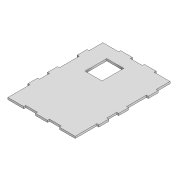
# Autodesk Inventor part: Sup´2
Saved by Autodesk Inventor 2022 (Build 260153000, 153)
## iProperties
Created: 2022-06-21
Part Number: Sup´2
Material: Generic
Document SubType Name: Modeling
Designer: ADMIN
Density: 1 g/cm^3
Appearance: Default
Author: ADMIN
Autodesk Inventor part; units mm, degrees
ref_plane "YZ Plane" through (0, 0, 0) normal (1, 0, 0) x (0, 1, 0)
ref_plane "XZ Plane" through (0, 0, 0) normal (0, 1, 0) x (-1, 0, 0)
ref_plane "XY Plane" through (0, 0, 0) normal (0, 0, 1) x (1, 0, 0)
sketch "Sketch1" plane through (0, 0, 0) normal (0, 1, 0) x (-1, 0, 0)
  line L0 (4.0305, 15.695) -> (174.0305, 15.695)
  line L1 (174.0305, 15.695) -> (174.0305, -224.305)
  line L2 (174.0305, -224.305) -> (4.0305, -224.305)
  line L3 (4.0305, -224.305) -> (4.0305, 15.695)
  line L4 (174.0305, -39.305) -> (169.0305, -39.305)
  line L5 (169.0305, -39.305) -> (169.0305, -64.305)
  line L6 (169.0305, -64.305) -> (174.0305, -64.305)
  line L7 (174.0305, -64.305) -> (174.0305, -39.305)
  line L8 (174.0305, -89.305) -> (169.0305, -89.305)
  line L9 (169.0305, -89.305) -> (169.0305, -114.305)
  line L10 (169.0305, -114.305) -> (174.0305, -114.305)
  line L11 (174.0305, -114.305) -> (174.0305, -89.305)
  line L12 (174.0305, -164.305) -> (169.0305, -164.305)
  line L13 (169.0305, -164.305) -> (169.0305, -189.305)
  line L14 (169.0305, -189.305) -> (174.0305, -189.305)
  line L15 (174.0305, -189.305) -> (174.0305, -164.305)
  line L16 (89.0305, 15.695) -> (89.0305, -224.305)
  line L17 (4.0305, -39.305) -> (9.0305, -39.305)
  line L18 (9.0305, -39.305) -> (9.0305, -64.305)
  line L19 (9.0305, -64.305) -> (4.0305, -64.305)
  line L20 (4.0305, -89.305) -> (9.0305, -89.305)
  line L21 (9.0305, -89.305) -> (9.0305, -114.305)
  line L22 (9.0305, -114.305) -> (4.0305, -114.305)
  line L23 (4.0305, -164.305) -> (9.0305, -164.305)
  line L24 (9.0305, -164.305) -> (9.0305, -189.305)
  line L25 (9.0305, -189.305) -> (4.0305, -189.305)
  line L26 (134.0305, 15.695) -> (104.0305, 15.695)
  line L27 (104.0305, 15.695) -> (104.0305, 10.695)
  line L28 (104.0305, 10.695) -> (134.0305, 10.695)
  line L29 (134.0305, 10.695) -> (134.0305, 15.695)
  line L30 (74.0305, 15.695) -> (44.0305, 15.695)
  line L31 (44.0305, 15.695) -> (44.0305, 10.695)
  line L32 (44.0305, 10.695) -> (74.0305, 10.695)
  line L33 (74.0305, 10.695) -> (74.0305, 15.695)
  line L34 (134.0305, -224.305) -> (104.0305, -224.305)
  line L35 (104.0305, -224.305) -> (104.0305, -219.305)
  line L36 (104.0305, -219.305) -> (134.0305, -219.305)
  line L37 (134.0305, -219.305) -> (134.0305, -224.305)
  line L38 (74.0305, -224.305) -> (44.0305, -224.305)
  line L39 (44.0305, -224.305) -> (44.0305, -219.305)
  line L40 (44.0305, -219.305) -> (74.0305, -219.305)
  line L41 (74.0305, -219.305) -> (74.0305, -224.305)
  line L42 (9.0305, -39.305) -> (-0.9695, -39.305)
  line L43 (-0.9695, -39.305) -> (-0.9695, -64.305)
  line L44 (-0.9695, -64.305) -> (9.0305, -64.305)
  line L45 (9.0305, -64.305) -> (9.0305, -39.305)
  line L46 (9.0305, -89.305) -> (-0.9695, -89.305)
  line L47 (-0.9695, -89.305) -> (-0.9695, -114.305)
  line L48 (-0.9695, -114.305) -> (9.0305, -114.305)
  line L49 (9.0305, -114.305) -> (9.0305, -89.305)
  line L50 (9.0305, -164.305) -> (-0.9695, -164.305)
  line L51 (-0.9695, -164.305) -> (-0.9695, -189.305)
  line L52 (-0.9695, -189.305) -> (9.0305, -189.305)
  line L53 (9.0305, -189.305) -> (9.0305, -164.305)
  line L54 (169.0305, -39.305) -> (179.0305, -39.305)
  line L55 (179.0305, -39.305) -> (179.0305, -64.305)
  line L56 (179.0305, -64.305) -> (169.0305, -64.305)
  line L57 (169.0305, -89.305) -> (179.0305, -89.305)
  line L58 (179.0305, -89.305) -> (179.0305, -114.305)
  line L59 (179.0305, -114.305) -> (169.0305, -114.305)
  line L60 (169.0305, -164.305) -> (179.0305, -164.305)
  line L61 (179.0305, -164.305) -> (179.0305, -189.305)
  line L62 (179.0305, -189.305) -> (169.0305, -189.305)
  line L63 (134.0305, -219.305) -> (104.0305, -219.305)
  line L64 (104.0305, -219.305) -> (104.0305, -229.305)
  line L65 (104.0305, -229.305) -> (134.0305, -229.305)
  line L66 (134.0305, -229.305) -> (134.0305, -219.305)
  line L67 (74.0305, -219.305) -> (44.0305, -219.305)
  line L68 (44.0305, -219.305) -> (44.0305, -229.305)
  line L69 (44.0305, -229.305) -> (74.0305, -229.305)
  line L70 (74.0305, -229.305) -> (74.0305, -219.305)
  point P0 (0, 0)
  dimension "d0" = 170
  dimension "d1" = 240
  dimension "d2" = 5
  dimension "d3" = 25
  dimension "d4" = 5
  dimension "d5" = 25
  dimension "d6" = 5
  dimension "d7" = 25
  dimension "d8" = 35
  dimension "d9" = 50
  dimension "d10" = 25
  dimension "d11" = 30
  dimension "d12" = 30
  dimension "d13" = 5
  dimension "d14" = 5
  dimension "d15" = 30
  dimension "d16" = 15
  dimension "d17" = 5
  dimension "d20" = 10
  dimension "d21" = 10
  dimension "d22" = 10
  constraints: 142 end point, 26 parallel, 21 symmetric about line, 13 horizontal, 13 perpendicular, 11 point on line, 2 midpoint
  measures "d0" distance of L1.end L2.end
  measures "d1" distance of L0.end L1.end
  measures "d2" distance of L6.end L5.end
  measures "d3" distance of L5.end L4.end
  measures "d4" distance of L10.end L9.end
  measures "d5" distance of L9.end L8.end
  measures "d6" distance of L14.end L13.end
  measures "d7" distance of L13.end L12.end
  measures "d8" distance between parallel lines of L2 L14
  measures "d9" distance between parallel lines of L10 L12
  measures "d10" distance between parallel lines of L6 L8
  measures "d11" distance of L28.end L27.end
  measures "d12" distance of L32.end L31.end
  measures "d13" distance of L31.end L30.end
  measures "d14" distance of L28.end L26.start
  measures "d15" distance between parallel lines of L33 L27
  measures "d16" distance between parallel lines of L16 L27
  measures "d17" distance of L34.end L35.end
  measures "d20" distance of L44.end L43.end
  measures "d21" distance of L48.end L47.end
  measures "d22" distance of L64.end L63.end
extrude "Extrusion1" add sketch "Sketch1" along normal blind 5 contours L0 L31 L32 L33 L16 L2 L41 L40 L39 L3 L25 L24 L23 L22 L21 L20 L19 L18 L17 | L17 L18 L19 L3 | L3 L44 L43 L42 | L0 L27 L28 L29 L1 L4 L5 L6 L8 L9 L10 L12 L13 L14 L2 L37 L36 L35 L16 | L20 L21 L22 L3 | L3 L48 L47 L46 | L35 L36 L37 L2 | L2 L66 L65 L64 | L70 L69 L68 L2 | L2 L39 L40 L41 | L23 L24 L25 L3 | L3 L52 L51 L50 | L54 L55 L56 L1 | L1 L6 L5 L4 | L14 L13 L12 L1 | L1 L60 L61 L62 | L57 L58 L59 L1 | L1 L10 L9 L8
sketch "Sketch2" plane through (0, 5, 0) normal (0, 1, 0) x (1, 0, 0)
  line L0 (-4.0305, 189.305) -> (-4.0305, 224.305) projected
  line L1 (-4.0305, 224.305) -> (-44.0305, 224.305) projected
  line L2 (-44.0305, 224.305) -> (-44.0305, 229.305) projected
  line L3 (-44.0305, 229.305) -> (-74.0305, 229.305) projected
  line L4 (-74.0305, 229.305) -> (-74.0305, 224.305) projected
  line L5 (-74.0305, 224.305) -> (-104.0305, 224.305) projected
  line L6 (-104.0305, 224.305) -> (-104.0305, 229.305) projected
  line L7 (-104.0305, 229.305) -> (-134.0305, 229.305) projected
  line L8 (-134.0305, 229.305) -> (-134.0305, 224.305) projected
  line L9 (-134.0305, 224.305) -> (-174.0305, 224.305) projected
  line L10 (-174.0305, 224.305) -> (-174.0305, 189.305) projected
  line L11 (-174.0305, 189.305) -> (-179.0305, 189.305) projected
  line L12 (-179.0305, 189.305) -> (-179.0305, 164.305) projected
  line L13 (-179.0305, 164.305) -> (-174.0305, 164.305) projected
  line L14 (-174.0305, 164.305) -> (-174.0305, 114.305) projected
  line L15 (-174.0305, 114.305) -> (-179.0305, 114.305) projected
  line L16 (-179.0305, 114.305) -> (-179.0305, 89.305) projected
  line L17 (-179.0305, 89.305) -> (-174.0305, 89.305) projected
  line L18 (-174.0305, 89.305) -> (-174.0305, 64.305) projected
  line L19 (-174.0305, 64.305) -> (-179.0305, 64.305) projected
  line L20 (-179.0305, 64.305) -> (-179.0305, 39.305) projected
  line L21 (-179.0305, 39.305) -> (-174.0305, 39.305) projected
  line L22 (-174.0305, 39.305) -> (-174.0305, -15.695) projected
  line L23 (-174.0305, -15.695) -> (-134.0305, -15.695) projected
  line L24 (-134.0305, -15.695) -> (-134.0305, -10.695) projected
  line L25 (-134.0305, -10.695) -> (-104.0305, -10.695) projected
  line L26 (-104.0305, -10.695) -> (-104.0305, -15.695) projected
  line L27 (-104.0305, -15.695) -> (-74.0305, -15.695) projected
  line L28 (-74.0305, -15.695) -> (-74.0305, -10.695) projected
  line L29 (-74.0305, -10.695) -> (-44.0305, -10.695) projected
  line L30 (-44.0305, -10.695) -> (-44.0305, -15.695) projected
  line L31 (-44.0305, -15.695) -> (-4.0305, -15.695) projected
  line L32 (-4.0305, -15.695) -> (-4.0305, 39.305) projected
  line L33 (-4.0305, 39.305) -> (0.9695, 39.305) projected
  line L34 (0.9695, 39.305) -> (0.9695, 64.305) projected
  line L35 (0.9695, 64.305) -> (-4.0305, 64.305) projected
  line L36 (-4.0305, 64.305) -> (-4.0305, 89.305) projected
  line L37 (-4.0305, 89.305) -> (0.9695, 89.305) projected
  line L38 (0.9695, 89.305) -> (0.9695, 114.305) projected
  line L39 (0.9695, 114.305) -> (-4.0305, 114.305) projected
  line L40 (-4.0305, 114.305) -> (-4.0305, 164.305) projected
  line L41 (-4.0305, 164.305) -> (0.9695, 164.305) projected
  line L42 (0.9695, 164.305) -> (0.9695, 189.305) projected
  line L43 (0.9695, 189.305) -> (-4.0305, 189.305) projected
  line L44 (-4.0305, 189.305) -> (-4.0305, 224.305) projected
  line L45 (-4.0305, 224.305) -> (-44.0305, 224.305) projected
  line L46 (-44.0305, 224.305) -> (-44.0305, 229.305) projected
  line L47 (-44.0305, 229.305) -> (-74.0305, 229.305) projected
  line L48 (-74.0305, 229.305) -> (-74.0305, 224.305) projected
  line L49 (-74.0305, 224.305) -> (-104.0305, 224.305) projected
  line L50 (-104.0305, 224.305) -> (-104.0305, 229.305) projected
  line L51 (-104.0305, 229.305) -> (-134.0305, 229.305) projected
  line L52 (-134.0305, 229.305) -> (-134.0305, 224.305) projected
  line L53 (-134.0305, 224.305) -> (-174.0305, 224.305) projected
  line L54 (-174.0305, 224.305) -> (-174.0305, 189.305) projected
  line L55 (-174.0305, 189.305) -> (-179.0305, 189.305) projected
  line L56 (-179.0305, 189.305) -> (-179.0305, 164.305) projected
  line L57 (-179.0305, 164.305) -> (-174.0305, 164.305) projected
  line L58 (-174.0305, 164.305) -> (-174.0305, 114.305) projected
  line L59 (-174.0305, 114.305) -> (-179.0305, 114.305) projected
  line L60 (-179.0305, 114.305) -> (-179.0305, 89.305) projected
  line L61 (-179.0305, 89.305) -> (-174.0305, 89.305) projected
  line L62 (-174.0305, 89.305) -> (-174.0305, 64.305) projected
  line L63 (-174.0305, 64.305) -> (-179.0305, 64.305) projected
  line L64 (-179.0305, 64.305) -> (-179.0305, 39.305) projected
  line L65 (-179.0305, 39.305) -> (-174.0305, 39.305) projected
  line L66 (-174.0305, 39.305) -> (-174.0305, -15.695) projected
  line L67 (-174.0305, -15.695) -> (-134.0305, -15.695) projected
  line L68 (-134.0305, -15.695) -> (-134.0305, -10.695) projected
  line L69 (-134.0305, -10.695) -> (-104.0305, -10.695) projected
  line L70 (-104.0305, -10.695) -> (-104.0305, -15.695) projected
  line L71 (-104.0305, -15.695) -> (-74.0305, -15.695) projected
  line L72 (-74.0305, -15.695) -> (-74.0305, -10.695) projected
  line L73 (-74.0305, -10.695) -> (-44.0305, -10.695) projected
  line L74 (-44.0305, -10.695) -> (-44.0305, -15.695) projected
  line L75 (-44.0305, -15.695) -> (-4.0305, -15.695) projected
  line L76 (-4.0305, -15.695) -> (-4.0305, 39.305) projected
  line L77 (-4.0305, 39.305) -> (0.9695, 39.305) projected
  line L78 (0.9695, 39.305) -> (0.9695, 64.305) projected
  line L79 (0.9695, 64.305) -> (-4.0305, 64.305) projected
  line L80 (-4.0305, 64.305) -> (-4.0305, 89.305) projected
  line L81 (-4.0305, 89.305) -> (0.9695, 89.305) projected
  line L82 (0.9695, 89.305) -> (0.9695, 114.305) projected
  line L83 (0.9695, 114.305) -> (-4.0305, 114.305) projected
  line L84 (-4.0305, 114.305) -> (-4.0305, 164.305) projected
  line L85 (-4.0305, 164.305) -> (0.9695, 164.305) projected
  line L86 (0.9695, 164.305) -> (0.9695, 189.305) projected
  line L87 (0.9695, 189.305) -> (-4.0305, 189.305) projected
  line L88 (-134.0305, 139.305) -> (-91.0305, 139.305)
  line L89 (-91.0305, 139.305) -> (-91.0305, 194.305)
  line L90 (-91.0305, 194.305) -> (-134.0305, 194.305)
  line L91 (-134.0305, 194.305) -> (-134.0305, 139.305)
  point P0 (0, 0)
  dimension "d23" = 55
  dimension "d24" = 43
  dimension "d25" = 40
  dimension "d26" = 30
  constraints: 8 end point, 2 parallel, 1 horizontal, 1 perpendicular
  measures "d23" distance of L90.end L88.start
  measures "d24" distance of L89.end L90.end
  measures "d25" distance between parallel lines of L91 L14
  measures "d26" distance between parallel lines of L9 L90
extrude "Extrusion3" cut sketch "Sketch2" against normal blind 5 contours L91 L90 L89 L88
equation "\"d16\" = 0.5 * d15"
body "Solid1"
